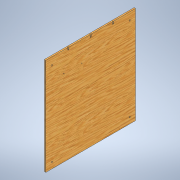
# Autodesk Inventor part: wallL2
Saved by Autodesk Inventor 2022 (Build 260153000, 153)
## iProperties
Created: 2022-02-21
Part Number: wallL2
Material: Plywood, Sheathing
Document SubType Name: Modeling
Designer: MarkP
Density: 0.552 g/cm^3
Appearance: Plywood - New
Author: MarkP
Autodesk Inventor part; units mm, degrees
ref_plane "YZ Plane" through (0, 0, 0) normal (1, 0, 0) x (0, 1, 0)
ref_plane "XZ Plane" through (0, 0, 0) normal (0, 1, 0) x (-1, 0, 0)
ref_plane "XY Plane" through (0, 0, 0) normal (0, 0, 1) x (1, 0, 0)
sketch "Sketch1" plane through (0, 0, 0) normal (1, 0, 0) x (0, 1, 0)
  line L0 (0, 0) -> (812, 0)
  line L1 (812, 0) -> (812, -750)
  line L2 (812, -750) -> (0, -750)
  line L3 (0, -750) -> (0, 0)
  dimension "d2" = 812
  dimension "d3" = 750
  constraints: 8 end point, 2 parallel, 1 horizontal, 1 perpendicular
  measures "d2" distance of L1.end L2.end
  measures "d3" distance of L0.end L1.end
extrude "Extrusion1" add sketch "Sketch1" along normal blind 12
sketch "Sketch2" plane through (12, 0, 0) normal (1, 0, 0) x (0, 0, -1)
  circle A0 centre (50, 50) radius 5
  circle A1 centre (700, 50) radius 5
  circle A2 centre (700, 750) radius 5
  circle A3 centre (50, 750) radius 5
  point P0 (0, 0)
  point P1 (750, 812)
  point P2 (750, 0)
  dimension "d15" = 10
  constraints: 4 centre point
  measures "d15" diameter of A2
extrude "Extrusion2" cut sketch "Sketch2" against normal blind 12
sketch "Sketch3" plane through (0, 812, 0) normal (0, 1, 0) x (1, 0, 0)
  line L0 (12, 375) -> (199, 375) construction
  circle A0 centre (12, 188) radius 5
  circle A1 centre (12, 375) radius 5
  circle A2 centre (12, 562) radius 5
  point P0 (0, 0)
  point P1 (12, 750)
  dimension "d23" = 10
  dimension "d24" = 10
  dimension "d25" = 10
  constraints: 3 centre point, 2 end point, 1 coincident, 1 horizontal
  measures "d23" diameter of A0
  measures "d24" diameter of A1
  measures "d25" diameter of A2
extrude "Extrusion3" cut sketch "Sketch3" against normal blind 20
sketch "Sketch4" plane through (0, 0, 0) normal (-1, 0, 0) x (0, 0, 1)
  circle A0 centre (-300, 640.75) radius 2.5
  circle A1 centre (-150, 640.75) radius 2.5
  point P0 (0, 812)
  constraints: 2 centre point
extrude "Extrusion4" cut sketch "Sketch4" against normal blind 20
body "Solid1"
